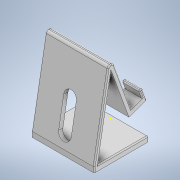
# Autodesk Inventor part: Phone Stand V3 Rev B
Saved by Autodesk Inventor 2021 (Build 250183000, 183)
## iProperties
Created: 2020-10-03
Part Number: Phone Stand V3 Rev B
Material: Generic
Document SubType Name: Modeling
Designer: cmzgt
Density: 1 g/cm^3
Appearance: Default
Author: cmzgt
Autodesk Inventor part; units mm, degrees
ref_plane "YZ Plane" through (0, 0, 0) normal (1, 0, 0) x (0, 1, 0)
ref_plane "XZ Plane" through (0, 0, 0) normal (0, 1, 0) x (-1, 0, 0)
ref_plane "XY Plane" through (0, 0, 0) normal (0, 0, 1) x (1, 0, 0)
sketch "Sketch1" plane through (0, 0, 0) normal (0, 1, 0) x (-1, 0, 0)
  line L0 (-38.1, -33.02) -> (38.1, -33.02)
  line L1 (38.1, -33.02) -> (38.1, 33.02)
  line L2 (38.1, 33.02) -> (-38.1, 33.02)
  line L3 (-38.1, 33.02) -> (-38.1, -33.02)
  line L4 (-38.1, -33.02) -> (38.1, 33.02) construction
  line L5 (38.1, -33.02) -> (-38.1, 33.02) construction
  point P0 (0, 0)
  dimension "d0" = 76.2
  dimension "d1" = 66.04
  constraints: 12 end point, 2 midpoint, 2 parallel, 1 horizontal, 1 perpendicular
  measures "d0" distance of L2.end L1.end
  measures "d1" distance of L1.end L0.end
extrude "Extrusion1" add sketch "Sketch1" along normal blind 6.35
sketch "Sketch3" plane through (38.1, 0, 33.02) normal (1, 0, 0) x (0, 0, -1)
  line L0 (66.04, 6.35) -> (0, 6.35) projected
  line L1 (0, 6.35) -> (6.35, 6.35) construction
  line L2 (0, 6.35) -> (17.2016, 103.9051)
  line L3 (17.2016, 103.9051) -> (23.6495, 103.9051)
  line L4 (23.6495, 103.9051) -> (47.1053, 39.4609)
  line L5 (47.1053, 39.4609) -> (42.3317, 37.7235)
  line L6 (42.3317, 37.7235) -> (21.0166, 96.2862)
  line L7 (21.0166, 96.2862) -> (5.1584, 6.35)
  point P0 (33.02, 0)
  dimension "d13" = 99.06
  dimension "d14" = 80
  dimension "d20" = 68.58
  dimension "d21" = 70
  dimension "d22" = 5.08
  dimension "d37" = 5.08
  constraints: 14 end point, 2 parallel, 2 point on line, 1 horizontal, 1 perpendicular
  measures "d13" distance of L0.end L2.end
  measures "d14" angle of L0 L2
  measures "d20" distance of L3.end L4.end
  measures "d21" angle of L0 L4
  measures "d22" distance of L4.end L5.end
  measures "d37" distance between parallel lines of L2 L7
extrude "Extrusion2" add sketch "Sketch3" against normal up to surface (76.2 mm away)
fillet "Fillet1" radius 3.175 2 edges at (0, 103.9051, 15.8184) (0, 103.9051, 9.3705)
sketch "Sketch6" plane through (38.1, 39.4609, -14.0853) normal (0, 0.3420201, -0.9396926) x (-1, 0, 0)
  line L0 (0, 0) -> (0, 66.3568) projected
  line L1 (0, 0) -> (21.59, 0)
  line L2 (21.59, 0) -> (21.59, 5.08)
  line L3 (21.59, 5.08) -> (0, 5.08)
  line L4 (0, 5.08) -> (0, 0)
  line L5 (0, 66.3568) -> (76.2, 66.3568) projected
  line L6 (38.1, 66.3568) -> (38.1, 0)
  line L7 (0, 0) -> (76.2, 0) projected
  line L8 (76.2, 0) -> (54.61, 0)
  line L9 (54.61, 0) -> (54.61, 5.08)
  line L10 (54.61, 5.08) -> (76.2, 5.08)
  line L11 (76.2, 0) -> (76.2, 66.3568) projected
  line L12 (76.2, 5.08) -> (76.2, 0)
  point P0 (38.1, -32.2637)
  point P1 (54.61, 0)
  point P2 (0, 5.08)
  dimension "d24" = 21.59
  dimension "d25" = 5.08
  constraints: 18 end point, 3 symmetric about line, 2 midpoint, 2 parallel, 1 collinear, 1 horizontal, 1 perpendicular
  measures "d24" distance of L3.end L2.end
  measures "d25" distance of L1.end L2.end
extrude "Extrusion3" add sketch "Sketch6" along normal blind 17.78 contours L0 L3 L2 L1 | L9 L10 L11 L7
sketch "Sketch7" plane through (16.51, 44.2346, -12.3478) normal (0, 0.9396926, 0.3420201) x (1, 0, 0)
  line L0 (0, 17.78) -> (21.59, 17.78) projected
  line L1 (21.59, 17.78) -> (0, 17.78)
  line L2 (0, 17.78) -> (0, 13.97)
  line L3 (0, 13.97) -> (21.59, 13.97)
  line L4 (21.59, 13.97) -> (21.59, 17.78)
  line L5 (21.59, -3.5556) -> (-54.61, -3.5556) projected
  line L6 (-16.51, -3.5556) -> (-16.51, 27.2379)
  line L7 (-33.02, 17.78) -> (-54.61, 17.78)
  line L8 (-33.02, 17.78) -> (-33.02, 13.97)
  line L9 (-33.02, 13.97) -> (-54.61, 13.97)
  line L10 (-54.61, 13.97) -> (-54.61, 17.78)
  line L11 (0, 0) -> (0, 17.78) projected
  point P0 (-16.51, -26.7323)
  dimension "d28" = 3.81
  constraints: 18 end point, 5 symmetric about line, 2 parallel, 1 horizontal, 1 midpoint, 1 perpendicular, 1 point on line, 1 vertical
  measures "d28" distance of L2.end L1.end
extrude "Extrusion4" add sketch "Sketch7" along normal blind 10.16
fillet "Fillet2" radius 1.27 19 edges at (38.1, 6.35, -2.5792) (0, 6.35, -33.02) (-38.1, 6.35, -2.5792) (-38.1, 3.175, -33.02) (38.1, 3.175, -33.02) (38.1, 3.175, 33.02) (-38.1, 3.175, 33.02) (-38.1, 103.1622, 15.1951) (-38.1, 103.9051, 12.3739) (-38.1, 103.3309, 9.7725) (-38.1, 73.0253, -1.8689) (-38.1, 53.8157, 24.6505) (-38.1, 51.3181, 19.9325) (38.1, 103.1622, 15.1951) (38.1, 103.9051, 12.3739) (38.1, 103.3309, 9.7725) (38.1, 73.0253, -1.8689) (38.1, 53.8157, 24.6505) (38.1, 51.3181, 19.9325)
fillet "Fillet3" radius 1.27 18 edges at (-38.1, 59.2114, -23.7905) (-27.305, 59.863, -25.5806) (-27.305, 58.5599, -22.0004) (-16.51, 59.2114, -23.7905) (16.51, 59.2114, -23.7905) (27.305, 59.863, -25.5806) (27.305, 58.5599, -22.0004) (38.1, 59.2114, -23.7905) (27.305, 45.5421, -30.793) (16.51, 52.7025, -28.1868) (38.1, 52.7025, -28.1868) (38.1, 53.7862, -23.7379) (-16.51, 53.7862, -23.7379) (-38.1, 53.7862, -23.7379) (-38.1, 52.7025, -28.1868) (-27.305, 45.5421, -30.793) (16.51, 53.7862, -23.7379) (-16.51, 52.7025, -28.1868)
sketch "Sketch9" plane through (-36.83, 6.35, 33.02) normal (0, 0.1736482, 0.9848078) x (1, 0, 0)
  line L0 (0, 0.8957) -> (73.66, 0.8957) construction
  line L1 (36.83, 0.8957) -> (36.83, 92.2194) construction
  line L2 (73.66, 92.2194) -> (0, 92.2194) construction
  line L3 (36.83, 15.1159) -> (36.83, 50.6759) construction
  line L4 (44.45, 15.1159) -> (44.45, 50.6759)
  line L5 (29.21, 50.6759) -> (29.21, 15.1159)
  arc A0 (29.21, 15.1159) -> (44.45, 15.1159) centre (36.83, 15.1159) ccw
  arc A1 (44.45, 50.6759) -> (29.21, 50.6759) centre (36.83, 50.6759) ccw
  line L6 (0, 96.3959) -> (73.66, 96.3959) projected
  point P0 (36.83, -0.5197)
  point P1 (36.83, 32.8959)
  dimension "d38" = 17.78
  dimension "d39" = 15.24
  dimension "d40" = 45.72
  constraints: 10 end point, 4 point on circle, 4 tangent, 3 midpoint, 2 centre point, 2 point on line, 1 parallel
  measures "d38" distance of point (36.83, 32.896) L3.end
  measures "d39" diameter of A1
  measures "d40" distance from line of L6 L3.end
extrude "Extrusion6" cut sketch "Sketch9" against normal up to next
sketch "Sketch10" plane through (16.51, 39.4609, -14.0853) normal (0, 0.3420201, -0.9396926) x (-1, 0, 0)
  point P0 (16.51, -32.2637)
body "Solid1"
